Autodesk Fusion 360 part; units mm, degrees
(part 9 of 14)
  line L5619 (-23.7596, 111.125) -> (-29.2589, 101.6)
  line L5620 (-29.2589, 101.6) -> (-23.7596, 92.075)
  line L5621 (-23.7596, 92.075) -> (-12.7611, 92.075)
  line L5622 (-7.2618, 101.6) -> (-12.7611, 111.125)
  line L5623 (-12.7611, 92.075) -> (-7.2618, 101.6)
  line L5624 (6.4863, 122.2375) -> (-4.5122, 122.2375)
  line L5625 (-4.5122, 122.2375) -> (-10.0114, 112.7125)
  line L5626 (-10.0114, 112.7125) -> (-4.5122, 103.1875)
  line L5627 (-4.5122, 103.1875) -> (6.4863, 103.1875)
  line L5628 (11.9856, 112.7125) -> (6.4863, 122.2375)
  line L5629 (6.4863, 103.1875) -> (11.9856, 112.7125)
  line L5630 (25.7337, 133.35) -> (14.7352, 133.35)
  line L5631 (14.7352, 133.35) -> (9.236, 123.825)
  line L5632 (9.236, 123.825) -> (14.7352, 114.3)
  line L5633 (14.7352, 114.3) -> (25.7337, 114.3)
  line L5634 (31.233, 123.825) -> (25.7337, 133.35)
  line L5635 (25.7337, 114.3) -> (31.233, 123.825)
  line L5636 (44.9812, 144.4625) -> (33.9826, 144.4625)
  line L5637 (33.9826, 144.4625) -> (28.4834, 134.9375)
  line L5638 (28.4834, 134.9375) -> (33.9826, 125.4125)
  line L5639 (33.9826, 125.4125) -> (44.9812, 125.4125)
  line L5640 (50.4804, 134.9375) -> (44.9812, 144.4625)
  line L5641 (44.9812, 125.4125) -> (50.4804, 134.9375)
  line L5642 (64.2286, 155.575) -> (53.2301, 155.575)
  line L5643 (53.2301, 155.575) -> (47.7308, 146.05)
  line L5644 (47.7308, 146.05) -> (53.2301, 136.525)
  line L5645 (53.2301, 136.525) -> (64.2286, 136.525)
  line L5646 (69.7278, 146.05) -> (64.2286, 155.575)
  line L5647 (64.2286, 136.525) -> (69.7278, 146.05)
  line L5648 (83.476, 166.6875) -> (72.4775, 166.6875)
  line L5649 (72.4775, 166.6875) -> (66.9782, 157.1625)
  line L5650 (66.9782, 157.1625) -> (72.4775, 147.6375)
  line L5651 (72.4775, 147.6375) -> (83.476, 147.6375)
  line L5652 (88.9753, 157.1625) -> (83.476, 166.6875)
  line L5653 (83.476, 147.6375) -> (88.9753, 157.1625)
  line L5654 (102.7234, 177.8) -> (91.7249, 177.8)
  line L5655 (91.7249, 177.8) -> (86.2256, 168.275)
  line L5656 (86.2256, 168.275) -> (91.7249, 158.75)
  line L5657 (91.7249, 158.75) -> (102.7234, 158.75)
  line L5658 (108.2227, 168.275) -> (102.7234, 177.8)
  line L5659 (102.7234, 158.75) -> (108.2227, 168.275)
  line L5660 (121.9708, 188.9125) -> (110.9723, 188.9125)
  line L5661 (110.9723, 188.9125) -> (105.473, 179.3875)
  line L5662 (105.473, 179.3875) -> (110.9723, 169.8625)
  line L5663 (110.9723, 169.8625) -> (121.9708, 169.8625)
  line L5664 (127.4701, 179.3875) -> (121.9708, 188.9125)
  line L5665 (121.9708, 169.8625) -> (127.4701, 179.3875)
  line L5666 (141.2182, 200.025) -> (130.2197, 200.025)
  line L5667 (130.2197, 200.025) -> (124.7205, 190.5)
  line L5668 (124.7205, 190.5) -> (130.2197, 180.975)
  line L5669 (130.2197, 180.975) -> (141.2182, 180.975)
  line L5670 (146.7175, 190.5) -> (141.2182, 200.025)
  line L5671 (141.2182, 180.975) -> (146.7175, 190.5)
  line L5672 (160.4657, 211.1375) -> (149.4671, 211.1375)
  line L5673 (149.4671, 211.1375) -> (143.9679, 201.6125)
  line L5674 (143.9679, 201.6125) -> (149.4671, 192.0875)
  line L5675 (149.4671, 192.0875) -> (160.4657, 192.0875)
  line L5676 (165.9649, 201.6125) -> (160.4657, 211.1375)
  line L5677 (160.4657, 192.0875) -> (165.9649, 201.6125)
  line L5678 (179.7131, 222.25) -> (168.7145, 222.25)
  line L5679 (168.7145, 222.25) -> (163.2153, 212.725)
  line L5680 (163.2153, 212.725) -> (168.7145, 203.2)
  line L5681 (168.7145, 203.2) -> (179.7131, 203.2)
  line L5682 (185.2123, 212.725) -> (179.7131, 222.25)
  line L5683 (179.7131, 203.2) -> (185.2123, 212.725)
  line L5684 (198.9605, 233.3625) -> (187.962, 233.3625)
  line L5685 (187.962, 233.3625) -> (182.4627, 223.8375)
  line L5686 (182.4627, 223.8375) -> (187.962, 214.3125)
  line L5687 (187.962, 214.3125) -> (198.9605, 214.3125)
  line L5688 (204.4597, 223.8375) -> (198.9605, 233.3625)
  line L5689 (198.9605, 214.3125) -> (204.4597, 223.8375)
  line L5690 (218.2079, 244.475) -> (207.2094, 244.475)
  line L5691 (207.2094, 244.475) -> (201.7101, 234.95)
  line L5692 (201.7101, 234.95) -> (207.2094, 225.425)
  line L5693 (207.2094, 225.425) -> (218.2079, 225.425)
  line L5694 (223.7072, 234.95) -> (218.2079, 244.475)
  line L5695 (218.2079, 225.425) -> (223.7072, 234.95)
  line L5696 (237.4553, 255.5875) -> (226.4568, 255.5875)
  line L5697 (226.4568, 255.5875) -> (220.9575, 246.0625)
  line L5698 (220.9575, 246.0625) -> (226.4568, 236.5375)
  line L5699 (226.4568, 236.5375) -> (237.4553, 236.5375)
  line L5700 (242.9546, 246.0625) -> (237.4553, 255.5875)
  line L5701 (237.4553, 236.5375) -> (242.9546, 246.0625)
  line L5702 (256.7027, 266.7) -> (245.7042, 266.7)
  line L5703 (245.7042, 266.7) -> (240.2049, 257.175)
  line L5704 (240.2049, 257.175) -> (245.7042, 247.65)
  line L5705 (245.7042, 247.65) -> (256.7027, 247.65)
  line L5706 (262.202, 257.175) -> (256.7027, 266.7)
  line L5707 (256.7027, 247.65) -> (262.202, 257.175)
  line L5708 (275.9501, 277.8125) -> (264.9516, 277.8125)
  line L5709 (264.9516, 277.8125) -> (259.4524, 268.2875)
  line L5710 (259.4524, 268.2875) -> (264.9516, 258.7625)
  line L5711 (264.9516, 258.7625) -> (275.9501, 258.7625)
  line L5712 (281.4494, 268.2875) -> (275.9501, 277.8125)
  line L5713 (275.9501, 258.7625) -> (281.4494, 268.2875)
  line L5714 (295.1976, 288.925) -> (284.199, 288.925)
  line L5715 (284.199, 288.925) -> (278.6998, 279.4)
  line L5716 (278.6998, 279.4) -> (284.199, 269.875)
  line L5717 (284.199, 269.875) -> (295.1976, 269.875)
  line L5718 (300.6968, 279.4) -> (295.1976, 288.925)
  line L5719 (295.1976, 269.875) -> (300.6968, 279.4)
  line L5720 (314.445, 300.0375) -> (303.4464, 300.0375)
  line L5721 (303.4464, 300.0375) -> (297.9472, 290.5125)
  line L5722 (297.9472, 290.5125) -> (303.4464, 280.9875)
  line L5723 (303.4464, 280.9875) -> (314.445, 280.9875)
  line L5724 (319.9442, 290.5125) -> (314.445, 300.0375)
  line L5725 (314.445, 280.9875) -> (319.9442, 290.5125)
  line L5726 (333.6924, 311.15) -> (322.6939, 311.15)
  line L5727 (322.6939, 311.15) -> (317.1946, 301.625)
  line L5728 (317.1946, 301.625) -> (322.6939, 292.1)
  line L5729 (322.6939, 292.1) -> (333.6924, 292.1)
  line L5730 (339.1916, 301.625) -> (333.6924, 311.15)
  line L5731 (333.6924, 292.1) -> (339.1916, 301.625)
  line L5732 (352.9398, 322.2625) -> (341.9413, 322.2625)
  line L5733 (341.9413, 322.2625) -> (336.442, 312.7375)
  line L5734 (336.442, 312.7375) -> (341.9413, 303.2125)
  line L5735 (341.9413, 303.2125) -> (352.9398, 303.2125)
  line L5736 (358.4391, 312.7375) -> (352.9398, 322.2625)
  line L5737 (352.9398, 303.2125) -> (358.4391, 312.7375)
  line L5738 (372.1872, 333.375) -> (361.1887, 333.375)
  line L5739 (361.1887, 333.375) -> (355.6894, 323.85)
  line L5740 (355.6894, 323.85) -> (361.1887, 314.325)
  line L5741 (361.1887, 314.325) -> (372.1872, 314.325)
  line L5742 (377.6865, 323.85) -> (372.1872, 333.375)
  line L5743 (372.1872, 314.325) -> (377.6865, 323.85)
  line L5744 (391.4346, 344.4875) -> (380.4361, 344.4875)
  line L5745 (380.4361, 344.4875) -> (374.9368, 334.9625)
  line L5746 (374.9368, 334.9625) -> (380.4361, 325.4375)
  line L5747 (380.4361, 325.4375) -> (391.4346, 325.4375)
  line L5748 (396.9339, 334.9625) -> (391.4346, 344.4875)
  line L5749 (391.4346, 325.4375) -> (396.9339, 334.9625)
  line L5750 (410.682, 355.6) -> (399.6835, 355.6)
  line L5751 (399.6835, 355.6) -> (394.1843, 346.075)
  line L5752 (394.1843, 346.075) -> (399.6835, 336.55)
  line L5753 (399.6835, 336.55) -> (410.682, 336.55)
  line L5754 (416.1813, 346.075) -> (410.682, 355.6)
  line L5755 (410.682, 336.55) -> (416.1813, 346.075)
  line L5756 (429.9295, 366.7125) -> (418.9309, 366.7125)
  line L5757 (418.9309, 366.7125) -> (413.4317, 357.1875)
  line L5758 (413.4317, 357.1875) -> (418.9309, 347.6625)
  line L5759 (418.9309, 347.6625) -> (429.9295, 347.6625)
  line L5760 (435.4287, 357.1875) -> (429.9295, 366.7125)
  line L5761 (429.9295, 347.6625) -> (435.4287, 357.1875)
  line L5762 (449.1769, 377.825) -> (438.1783, 377.825)
  line L5763 (438.1783, 377.825) -> (432.6791, 368.3)
  line L5764 (432.6791, 368.3) -> (438.1783, 358.775)
  line L5765 (438.1783, 358.775) -> (449.1769, 358.775)
  line L5766 (454.6761, 368.3) -> (449.1769, 377.825)
  line L5767 (449.1769, 358.775) -> (454.6761, 368.3)
  line L5768 (468.4243, 388.9375) -> (457.4258, 388.9375)
  line L5769 (457.4258, 388.9375) -> (451.9265, 379.4125)
  line L5770 (451.9265, 379.4125) -> (457.4258, 369.8875)
  line L5771 (457.4258, 369.8875) -> (468.4243, 369.8875)
  line L5772 (473.9235, 379.4125) -> (468.4243, 388.9375)
  line L5773 (468.4243, 369.8875) -> (473.9235, 379.4125)
  line L5774 (-686.4206, -255.5875) -> (-697.4191, -255.5875)
  line L5775 (-697.4191, -255.5875) -> (-702.9184, -265.1125)
  line L5776 (-702.9184, -265.1125) -> (-697.4191, -274.6375)
  line L5777 (-697.4191, -274.6375) -> (-686.4206, -274.6375)
  line L5778 (-680.9213, -265.1125) -> (-686.4206, -255.5875)
  line L5779 (-686.4206, -274.6375) -> (-680.9213, -265.1125)
  line L5780 (-667.1732, -244.475) -> (-678.1717, -244.475)
  line L5781 (-678.1717, -244.475) -> (-683.671, -254)
  line L5782 (-683.671, -254) -> (-678.1717, -263.525)
  line L5783 (-678.1717, -263.525) -> (-667.1732, -263.525)
  line L5784 (-661.6739, -254) -> (-667.1732, -244.475)
  line L5785 (-667.1732, -263.525) -> (-661.6739, -254)
  line L5786 (-647.9258, -233.3625) -> (-658.9243, -233.3625)
  line L5787 (-658.9243, -233.3625) -> (-664.4235, -242.8875)
  line L5788 (-664.4235, -242.8875) -> (-658.9243, -252.4125)
  line L5789 (-658.9243, -252.4125) -> (-647.9258, -252.4125)
  line L5790 (-642.4265, -242.8875) -> (-647.9258, -233.3625)
  line L5791 (-647.9258, -252.4125) -> (-642.4265, -242.8875)
  line L5792 (-628.6783, -222.25) -> (-639.6769, -222.25)
  line L5793 (-639.6769, -222.25) -> (-645.1761, -231.775)
  line L5794 (-645.1761, -231.775) -> (-639.6769, -241.3)
  line L5795 (-639.6769, -241.3) -> (-628.6783, -241.3)
  line L5796 (-623.1791, -231.775) -> (-628.6783, -222.25)
  line L5797 (-628.6783, -241.3) -> (-623.1791, -231.775)
  line L5798 (-609.4309, -211.1375) -> (-620.4295, -211.1375)
  line L5799 (-620.4295, -211.1375) -> (-625.9287, -220.6625)
  line L5800 (-625.9287, -220.6625) -> (-620.4295, -230.1875)
  line L5801 (-620.4295, -230.1875) -> (-609.4309, -230.1875)
  line L5802 (-603.9317, -220.6625) -> (-609.4309, -211.1375)
  line L5803 (-609.4309, -230.1875) -> (-603.9317, -220.6625)
  line L5804 (-590.1835, -200.025) -> (-601.182, -200.025)
  line L5805 (-601.182, -200.025) -> (-606.6813, -209.55)
  line L5806 (-606.6813, -209.55) -> (-601.182, -219.075)
  line L5807 (-601.182, -219.075) -> (-590.1835, -219.075)
  line L5808 (-584.6843, -209.55) -> (-590.1835, -200.025)
  line L5809 (-590.1835, -219.075) -> (-584.6843, -209.55)
  line L5810 (-570.9361, -188.9125) -> (-581.9346, -188.9125)
  line L5811 (-581.9346, -188.9125) -> (-587.4339, -198.4375)
  line L5812 (-587.4339, -198.4375) -> (-581.9346, -207.9625)
  line L5813 (-581.9346, -207.9625) -> (-570.9361, -207.9625)
  line L5814 (-565.4368, -198.4375) -> (-570.9361, -188.9125)
  line L5815 (-570.9361, -207.9625) -> (-565.4368, -198.4375)
  line L5816 (-551.6887, -177.8) -> (-562.6872, -177.8)
  line L5817 (-562.6872, -177.8) -> (-568.1865, -187.325)
  line L5818 (-568.1865, -187.325) -> (-562.6872, -196.85)
  line L5819 (-562.6872, -196.85) -> (-551.6887, -196.85)
  line L5820 (-546.1894, -187.325) -> (-551.6887, -177.8)
  line L5821 (-551.6887, -196.85) -> (-546.1894, -187.325)
  line L5822 (-532.4413, -166.6875) -> (-543.4398, -166.6875)
  line L5823 (-543.4398, -166.6875) -> (-548.9391, -176.2125)
  line L5824 (-548.9391, -176.2125) -> (-543.4398, -185.7375)
  line L5825 (-543.4398, -185.7375) -> (-532.4413, -185.7375)
  line L5826 (-526.942, -176.2125) -> (-532.4413, -166.6875)
  line L5827 (-532.4413, -185.7375) -> (-526.942, -176.2125)
  line L5828 (-513.1939, -155.575) -> (-524.1924, -155.575)
  line L5829 (-524.1924, -155.575) -> (-529.6916, -165.1)
  line L5830 (-529.6916, -165.1) -> (-524.1924, -174.625)
  line L5831 (-524.1924, -174.625) -> (-513.1939, -174.625)
  line L5832 (-507.6946, -165.1) -> (-513.1939, -155.575)
  line L5833 (-513.1939, -174.625) -> (-507.6946, -165.1)
  line L5834 (-493.9464, -144.4625) -> (-504.945, -144.4625)
  line L5835 (-504.945, -144.4625) -> (-510.4442, -153.9875)
  line L5836 (-510.4442, -153.9875) -> (-504.945, -163.5125)
  line L5837 (-504.945, -163.5125) -> (-493.9464, -163.5125)
  line L5838 (-488.4472, -153.9875) -> (-493.9464, -144.4625)
  line L5839 (-493.9464, -163.5125) -> (-488.4472, -153.9875)
  line L5840 (-474.699, -133.35) -> (-485.6976, -133.35)
  line L5841 (-485.6976, -133.35) -> (-491.1968, -142.875)
  line L5842 (-491.1968, -142.875) -> (-485.6976, -152.4)
  line L5843 (-485.6976, -152.4) -> (-474.699, -152.4)
  line L5844 (-469.1998, -142.875) -> (-474.699, -133.35)
  line L5845 (-474.699, -152.4) -> (-469.1998, -142.875)
  line L5846 (-455.4516, -122.2375) -> (-466.4501, -122.2375)
  line L5847 (-466.4501, -122.2375) -> (-471.9494, -131.7625)
  line L5848 (-471.9494, -131.7625) -> (-466.4501, -141.2875)
  line L5849 (-466.4501, -141.2875) -> (-455.4516, -141.2875)
  line L5850 (-449.9524, -131.7625) -> (-455.4516, -122.2375)
  line L5851 (-455.4516, -141.2875) -> (-449.9524, -131.7625)
  line L5852 (-436.2042, -111.125) -> (-447.2027, -111.125)
  line L5853 (-447.2027, -111.125) -> (-452.702, -120.65)
  line L5854 (-452.702, -120.65) -> (-447.2027, -130.175)
  line L5855 (-447.2027, -130.175) -> (-436.2042, -130.175)
  line L5856 (-430.7049, -120.65) -> (-436.2042, -111.125)
  line L5857 (-436.2042, -130.175) -> (-430.7049, -120.65)
  line L5858 (-416.9568, -100.0125) -> (-427.9553, -100.0125)
  line L5859 (-427.9553, -100.0125) -> (-433.4546, -109.5375)
  line L5860 (-433.4546, -109.5375) -> (-427.9553, -119.0625)
  line L5861 (-427.9553, -119.0625) -> (-416.9568, -119.0625)
  line L5862 (-411.4575, -109.5375) -> (-416.9568, -100.0125)
  line L5863 (-416.9568, -119.0625) -> (-411.4575, -109.5375)
  line L5864 (-397.7094, -88.9) -> (-408.7079, -88.9)
  line L5865 (-408.7079, -88.9) -> (-414.2072, -98.425)
  line L5866 (-414.2072, -98.425) -> (-408.7079, -107.95)
  line L5867 (-408.7079, -107.95) -> (-397.7094, -107.95)
  line L5868 (-392.2101, -98.425) -> (-397.7094, -88.9)
  line L5869 (-397.7094, -107.95) -> (-392.2101, -98.425)
  line L5870 (-378.462, -77.7875) -> (-389.4605, -77.7875)
  line L5871 (-389.4605, -77.7875) -> (-394.9597, -87.3125)
  line L5872 (-394.9597, -87.3125) -> (-389.4605, -96.8375)
  line L5873 (-389.4605, -96.8375) -> (-378.462, -96.8375)
  line L5874 (-372.9627, -87.3125) -> (-378.462, -77.7875)
  line L5875 (-378.462, -96.8375) -> (-372.9627, -87.3125)
  line L5876 (-359.2145, -66.675) -> (-370.2131, -66.675)
  line L5877 (-370.2131, -66.675) -> (-375.7123, -76.2)
  line L5878 (-375.7123, -76.2) -> (-370.2131, -85.725)
  line L5879 (-370.2131, -85.725) -> (-359.2145, -85.725)
  line L5880 (-353.7153, -76.2) -> (-359.2145, -66.675)
  line L5881 (-359.2145, -85.725) -> (-353.7153, -76.2)
  line L5882 (-339.9671, -55.5625) -> (-350.9657, -55.5625)
  line L5883 (-350.9657, -55.5625) -> (-356.4649, -65.0875)
  line L5884 (-356.4649, -65.0875) -> (-350.9657, -74.6125)
  line L5885 (-350.9657, -74.6125) -> (-339.9671, -74.6125)
  line L5886 (-334.4679, -65.0875) -> (-339.9671, -55.5625)
  line L5887 (-339.9671, -74.6125) -> (-334.4679, -65.0875)
  line L5888 (-320.7197, -44.45) -> (-331.7182, -44.45)
  line L5889 (-331.7182, -44.45) -> (-337.2175, -53.975)
  line L5890 (-337.2175, -53.975) -> (-331.7182, -63.5)
  line L5891 (-331.7182, -63.5) -> (-320.7197, -63.5)
  line L5892 (-315.2205, -53.975) -> (-320.7197, -44.45)
  line L5893 (-320.7197, -63.5) -> (-315.2205, -53.975)
  line L5894 (-301.4723, -33.3375) -> (-312.4708, -33.3375)
  line L5895 (-312.4708, -33.3375) -> (-317.9701, -42.8625)
  line L5896 (-317.9701, -42.8625) -> (-312.4708, -52.3875)
  line L5897 (-312.4708, -52.3875) -> (-301.4723, -52.3875)
  line L5898 (-295.973, -42.8625) -> (-301.4723, -33.3375)
  line L5899 (-301.4723, -52.3875) -> (-295.973, -42.8625)
  line L5900 (-282.2249, -22.225) -> (-293.2234, -22.225)
  line L5901 (-293.2234, -22.225) -> (-298.7227, -31.75)
  line L5902 (-298.7227, -31.75) -> (-293.2234, -41.275)
  line L5903 (-293.2234, -41.275) -> (-282.2249, -41.275)
  line L5904 (-276.7256, -31.75) -> (-282.2249, -22.225)
  line L5905 (-282.2249, -41.275) -> (-276.7256, -31.75)
  line L5906 (-262.9775, -11.1125) -> (-273.976, -11.1125)
  line L5907 (-273.976, -11.1125) -> (-279.4753, -20.6375)
  line L5908 (-279.4753, -20.6375) -> (-273.976, -30.1625)
  line L5909 (-273.976, -30.1625) -> (-262.9775, -30.1625)
  line L5910 (-257.4782, -20.6375) -> (-262.9775, -11.1125)
  line L5911 (-262.9775, -30.1625) -> (-257.4782, -20.6375)
  line L5912 (-243.7301, 0) -> (-254.7286, 0)
  line L5913 (-254.7286, 0) -> (-260.2278, -9.525)
  line L5914 (-260.2278, -9.525) -> (-254.7286, -19.05)
  line L5915 (-254.7286, -19.05) -> (-243.7301, -19.05)
  line L5916 (-238.2308, -9.525) -> (-243.7301, 0)
  line L5917 (-243.7301, -19.05) -> (-238.2308, -9.525)
  line L5918 (-224.4826, 11.1125) -> (-235.4812, 11.1125)
  line L5919 (-235.4812, 11.1125) -> (-240.9804, 1.5875)
  line L5920 (-240.9804, 1.5875) -> (-235.4812, -7.9375)
  line L5921 (-235.4812, -7.9375) -> (-224.4826, -7.9375)
  line L5922 (-218.9834, 1.5875) -> (-224.4826, 11.1125)
  line L5923 (-224.4826, -7.9375) -> (-218.9834, 1.5875)
  line L5924 (-205.2352, 22.225) -> (-216.2337, 22.225)
  line L5925 (-216.2337, 22.225) -> (-221.733, 12.7)
  line L5926 (-221.733, 12.7) -> (-216.2337, 3.175)
  line L5927 (-216.2337, 3.175) -> (-205.2352, 3.175)
  line L5928 (-199.736, 12.7) -> (-205.2352, 22.225)
  line L5929 (-205.2352, 3.175) -> (-199.736, 12.7)
  line L5930 (-185.9878, 33.3375) -> (-196.9863, 33.3375)
  line L5931 (-196.9863, 33.3375) -> (-202.4856, 23.8125)
  line L5932 (-202.4856, 23.8125) -> (-196.9863, 14.2875)
  line L5933 (-196.9863, 14.2875) -> (-185.9878, 14.2875)
  line L5934 (-180.4886, 23.8125) -> (-185.9878, 33.3375)
  line L5935 (-185.9878, 14.2875) -> (-180.4886, 23.8125)
  line L5936 (-166.7404, 44.45) -> (-177.7389, 44.45)
  line L5937 (-177.7389, 44.45) -> (-183.2382, 34.925)
  line L5938 (-183.2382, 34.925) -> (-177.7389, 25.4)
  line L5939 (-177.7389, 25.4) -> (-166.7404, 25.4)
  line L5940 (-161.2411, 34.925) -> (-166.7404, 44.45)
  line L5941 (-166.7404, 25.4) -> (-161.2411, 34.925)
  line L5942 (-147.493, 55.5625) -> (-158.4915, 55.5625)
  line L5943 (-158.4915, 55.5625) -> (-163.9908, 46.0375)
  line L5944 (-163.9908, 46.0375) -> (-158.4915, 36.5125)
  line L5945 (-158.4915, 36.5125) -> (-147.493, 36.5125)
  line L5946 (-141.9937, 46.0375) -> (-147.493, 55.5625)
  line L5947 (-147.493, 36.5125) -> (-141.9937, 46.0375)
  line L5948 (-128.2456, 66.675) -> (-139.2441, 66.675)
  line L5949 (-139.2441, 66.675) -> (-144.7434, 57.15)
  line L5950 (-144.7434, 57.15) -> (-139.2441, 47.625)
  line L5951 (-139.2441, 47.625) -> (-128.2456, 47.625)
  line L5952 (-122.7463, 57.15) -> (-128.2456, 66.675)
  line L5953 (-128.2456, 47.625) -> (-122.7463, 57.15)
  line L5954 (-108.9982, 77.7875) -> (-119.9967, 77.7875)
  line L5955 (-119.9967, 77.7875) -> (-125.4959, 68.2625)
  line L5956 (-125.4959, 68.2625) -> (-119.9967, 58.7375)
  line L5957 (-119.9967, 58.7375) -> (-108.9982, 58.7375)
  line L5958 (-103.4989, 68.2625) -> (-108.9982, 77.7875)
  line L5959 (-108.9982, 58.7375) -> (-103.4989, 68.2625)
  line L5960 (-89.7507, 88.9) -> (-100.7493, 88.9)
  line L5961 (-100.7493, 88.9) -> (-106.2485, 79.375)
  line L5962 (-106.2485, 79.375) -> (-100.7493, 69.85)
  line L5963 (-100.7493, 69.85) -> (-89.7507, 69.85)
  line L5964 (-84.2515, 79.375) -> (-89.7507, 88.9)
  line L5965 (-89.7507, 69.85) -> (-84.2515, 79.375)
  line L5966 (-70.5033, 100.0125) -> (-81.5018, 100.0125)
  line L5967 (-81.5018, 100.0125) -> (-87.0011, 90.4875)
  line L5968 (-87.0011, 90.4875) -> (-81.5018, 80.9625)
  line L5969 (-81.5018, 80.9625) -> (-70.5033, 80.9625)
  line L5970 (-65.0041, 90.4875) -> (-70.5033, 100.0125)
  line L5971 (-70.5033, 80.9625) -> (-65.0041, 90.4875)
  line L5972 (-51.2559, 111.125) -> (-62.2544, 111.125)
  line L5973 (-62.2544, 111.125) -> (-67.7537, 101.6)
  line L5974 (-67.7537, 101.6) -> (-62.2544, 92.075)
  line L5975 (-62.2544, 92.075) -> (-51.2559, 92.075)
  line L5976 (-45.7566, 101.6) -> (-51.2559, 111.125)
  line L5977 (-51.2559, 92.075) -> (-45.7566, 101.6)
  line L5978 (-32.0085, 122.2375) -> (-43.007, 122.2375)
  line L5979 (-43.007, 122.2375) -> (-48.5063, 112.7125)
  line L5980 (-48.5063, 112.7125) -> (-43.007, 103.1875)
  line L5981 (-43.007, 103.1875) -> (-32.0085, 103.1875)
  line L5982 (-26.5092, 112.7125) -> (-32.0085, 122.2375)
  line L5983 (-32.0085, 103.1875) -> (-26.5092, 112.7125)
  line L5984 (-12.7611, 133.35) -> (-23.7596, 133.35)
  line L5985 (-23.7596, 133.35) -> (-29.2589, 123.825)
  line L5986 (-29.2589, 123.825) -> (-23.7596, 114.3)
  line L5987 (-23.7596, 114.3) -> (-12.7611, 114.3)
  line L5988 (-7.2618, 123.825) -> (-12.7611, 133.35)
  line L5989 (-12.7611, 114.3) -> (-7.2618, 123.825)
  line L5990 (6.4863, 144.4625) -> (-4.5122, 144.4625)
  line L5991 (-4.5122, 144.4625) -> (-10.0114, 134.9375)
  line L5992 (-10.0114, 134.9375) -> (-4.5122, 125.4125)
  line L5993 (-4.5122, 125.4125) -> (6.4863, 125.4125)
  line L5994 (11.9856, 134.9375) -> (6.4863, 144.4625)
  line L5995 (6.4863, 125.4125) -> (11.9856, 134.9375)
  line L5996 (25.7337, 155.575) -> (14.7352, 155.575)
  line L5997 (14.7352, 155.575) -> (9.236, 146.05)
  line L5998 (9.236, 146.05) -> (14.7352, 136.525)
  line L5999 (14.7352, 136.525) -> (25.7337, 136.525)
  line L6000 (31.233, 146.05) -> (25.7337, 155.575)
  line L6001 (25.7337, 136.525) -> (31.233, 146.05)
  line L6002 (44.9812, 166.6875) -> (33.9826, 166.6875)
  line L6003 (33.9826, 166.6875) -> (28.4834, 157.1625)
  line L6004 (28.4834, 157.1625) -> (33.9826, 147.6375)
  line L6005 (33.9826, 147.6375) -> (44.9812, 147.6375)
  line L6006 (50.4804, 157.1625) -> (44.9812, 166.6875)
  line L6007 (44.9812, 147.6375) -> (50.4804, 157.1625)
  line L6008 (64.2286, 177.8) -> (53.2301, 177.8)
  line L6009 (53.2301, 177.8) -> (47.7308, 168.275)
  line L6010 (47.7308, 168.275) -> (53.2301, 158.75)
  line L6011 (53.2301, 158.75) -> (64.2286, 158.75)
  line L6012 (69.7278, 168.275) -> (64.2286, 177.8)
  line L6013 (64.2286, 158.75) -> (69.7278, 168.275)
  line L6014 (83.476, 188.9125) -> (72.4775, 188.9125)
  line L6015 (72.4775, 188.9125) -> (66.9782, 179.3875)
  line L6016 (66.9782, 179.3875) -> (72.4775, 169.8625)
  line L6017 (72.4775, 169.8625) -> (83.476, 169.8625)
  line L6018 (88.9753, 179.3875) -> (83.476, 188.9125)
  line L6019 (83.476, 169.8625) -> (88.9753, 179.3875)
  line L6020 (102.7234, 200.025) -> (91.7249, 200.025)
  line L6021 (91.7249, 200.025) -> (86.2256, 190.5)
  line L6022 (86.2256, 190.5) -> (91.7249, 180.975)
  line L6023 (91.7249, 180.975) -> (102.7234, 180.975)
  line L6024 (108.2227, 190.5) -> (102.7234, 200.025)
  line L6025 (102.7234, 180.975) -> (108.2227, 190.5)
  line L6026 (121.9708, 211.1375) -> (110.9723, 211.1375)
  line L6027 (110.9723, 211.1375) -> (105.473, 201.6125)
  line L6028 (105.473, 201.6125) -> (110.9723, 192.0875)
  line L6029 (110.9723, 192.0875) -> (121.9708, 192.0875)
  line L6030 (127.4701, 201.6125) -> (121.9708, 211.1375)
  line L6031 (121.9708, 192.0875) -> (127.4701, 201.6125)
  line L6032 (141.2182, 222.25) -> (130.2197, 222.25)
  line L6033 (130.2197, 222.25) -> (124.7205, 212.725)
  line L6034 (124.7205, 212.725) -> (130.2197, 203.2)
  line L6035 (130.2197, 203.2) -> (141.2182, 203.2)
  line L6036 (146.7175, 212.725) -> (141.2182, 222.25)
  line L6037 (141.2182, 203.2) -> (146.7175, 212.725)
  line L6038 (160.4657, 233.3625) -> (149.4671, 233.3625)
  line L6039 (149.4671, 233.3625) -> (143.9679, 223.8375)
  line L6040 (143.9679, 223.8375) -> (149.4671, 214.3125)
  line L6041 (149.4671, 214.3125) -> (160.4657, 214.3125)
  line L6042 (165.9649, 223.8375) -> (160.4657, 233.3625)
  line L6043 (160.4657, 214.3125) -> (165.9649, 223.8375)
  line L6044 (179.7131, 244.475) -> (168.7145, 244.475)
  line L6045 (168.7145, 244.475) -> (163.2153, 234.95)
  line L6046 (163.2153, 234.95) -> (168.7145, 225.425)
  line L6047 (168.7145, 225.425) -> (179.7131, 225.425)
  line L6048 (185.2123, 234.95) -> (179.7131, 244.475)
  line L6049 (179.7131, 225.425) -> (185.2123, 234.95)
  line L6050 (198.9605, 255.5875) -> (187.962, 255.5875)
  line L6051 (187.962, 255.5875) -> (182.4627, 246.0625)
  line L6052 (182.4627, 246.0625) -> (187.962, 236.5375)
  line L6053 (187.962, 236.5375) -> (198.9605, 236.5375)
  line L6054 (204.4597, 246.0625) -> (198.9605, 255.5875)
  line L6055 (198.9605, 236.5375) -> (204.4597, 246.0625)
  line L6056 (218.2079, 266.7) -> (207.2094, 266.7)
  line L6057 (207.2094, 266.7) -> (201.7101, 257.175)
  line L6058 (201.7101, 257.175) -> (207.2094, 247.65)
  line L6059 (207.2094, 247.65) -> (218.2079, 247.65)
  line L6060 (223.7072, 257.175) -> (218.2079, 266.7)
  line L6061 (218.2079, 247.65) -> (223.7072, 257.175)
  line L6062 (237.4553, 277.8125) -> (226.4568, 277.8125)
  line L6063 (226.4568, 277.8125) -> (220.9575, 268.2875)
  line L6064 (220.9575, 268.2875) -> (226.4568, 258.7625)
  line L6065 (226.4568, 258.7625) -> (237.4553, 258.7625)
  line L6066 (242.9546, 268.2875) -> (237.4553, 277.8125)
  line L6067 (237.4553, 258.7625) -> (242.9546, 268.2875)
  line L6068 (256.7027, 288.925) -> (245.7042, 288.925)
  line L6069 (245.7042, 288.925) -> (240.2049, 279.4)
  line L6070 (240.2049, 279.4) -> (245.7042, 269.875)
  line L6071 (245.7042, 269.875) -> (256.7027, 269.875)
  line L6072 (262.202, 279.4) -> (256.7027, 288.925)
  line L6073 (256.7027, 269.875) -> (262.202, 279.4)
  line L6074 (275.9501, 300.0375) -> (264.9516, 300.0375)
  line L6075 (264.9516, 300.0375) -> (259.4524, 290.5125)
  line L6076 (259.4524, 290.5125) -> (264.9516, 280.9875)
  line L6077 (264.9516, 280.9875) -> (275.9501, 280.9875)
  line L6078 (281.4494, 290.5125) -> (275.9501, 300.0375)
  line L6079 (275.9501, 280.9875) -> (281.4494, 290.5125)
  line L6080 (295.1976, 311.15) -> (284.199, 311.15)
  line L6081 (284.199, 311.15) -> (278.6998, 301.625)
  line L6082 (278.6998, 301.625) -> (284.199, 292.1)
  line L6083 (284.199, 292.1) -> (295.1976, 292.1)
  line L6084 (300.6968, 301.625) -> (295.1976, 311.15)
  line L6085 (295.1976, 292.1) -> (300.6968, 301.625)
  line L6086 (314.445, 322.2625) -> (303.4464, 322.2625)
  line L6087 (303.4464, 322.2625) -> (297.9472, 312.7375)
  line L6088 (297.9472, 312.7375) -> (303.4464, 303.2125)
  line L6089 (303.4464, 303.2125) -> (314.445, 303.2125)
  line L6090 (319.9442, 312.7375) -> (314.445, 322.2625)
  line L6091 (314.445, 303.2125) -> (319.9442, 312.7375)
  line L6092 (333.6924, 333.375) -> (322.6939, 333.375)
  line L6093 (322.6939, 333.375) -> (317.1946, 323.85)
  line L6094 (317.1946, 323.85) -> (322.6939, 314.325)
  line L6095 (322.6939, 314.325) -> (333.6924, 314.325)
  line L6096 (339.1916, 323.85) -> (333.6924, 333.375)
  line L6097 (333.6924, 314.325) -> (339.1916, 323.85)
  line L6098 (352.9398, 344.4875) -> (341.9413, 344.4875)
  line L6099 (341.9413, 344.4875) -> (336.442, 334.9625)
  line L6100 (336.442, 334.9625) -> (341.9413, 325.4375)
  line L6101 (341.9413, 325.4375) -> (352.9398, 325.4375)
  line L6102 (358.4391, 334.9625) -> (352.9398, 344.4875)
  line L6103 (352.9398, 325.4375) -> (358.4391, 334.9625)
  line L6104 (372.1872, 355.6) -> (361.1887, 355.6)
  line L6105 (361.1887, 355.6) -> (355.6894, 346.075)
  line L6106 (355.6894, 346.075) -> (361.1887, 336.55)
  line L6107 (361.1887, 336.55) -> (372.1872, 336.55)
  line L6108 (377.6865, 346.075) -> (372.1872, 355.6)
  line L6109 (372.1872, 336.55) -> (377.6865, 346.075)
  line L6110 (391.4346, 366.7125) -> (380.4361, 366.7125)
  line L6111 (380.4361, 366.7125) -> (374.9368, 357.1875)
  line L6112 (374.9368, 357.1875) -> (380.4361, 347.6625)
  line L6113 (380.4361, 347.6625) -> (391.4346, 347.6625)
  line L6114 (396.9339, 357.1875) -> (391.4346, 366.7125)
  line L6115 (391.4346, 347.6625) -> (396.9339, 357.1875)
  line L6116 (410.682, 377.825) -> (399.6835, 377.825)
  line L6117 (399.6835, 377.825) -> (394.1843, 368.3)
  line L6118 (394.1843, 368.3) -> (399.6835, 358.775)
  line L6119 (399.6835, 358.775) -> (410.682, 358.775)
  line L6120 (416.1813, 368.3) -> (410.682, 377.825)
  line L6121 (410.682, 358.775) -> (416.1813, 368.3)
  line L6122 (429.9295, 388.9375) -> (418.9309, 388.9375)
  line L6123 (418.9309, 388.9375) -> (413.4317, 379.4125)
  line L6124 (413.4317, 379.4125) -> (418.9309, 369.8875)
  line L6125 (418.9309, 369.8875) -> (429.9295, 369.8875)
  line L6126 (435.4287, 379.4125) -> (429.9295, 388.9375)
  line L6127 (429.9295, 369.8875) -> (435.4287, 379.4125)
  line L6128 (449.1769, 400.05) -> (438.1783, 400.05)
  line L6129 (438.1783, 400.05) -> (432.6791, 390.525)
  line L6130 (432.6791, 390.525) -> (438.1783, 381)
  line L6131 (438.1783, 381) -> (449.1769, 381)
  line L6132 (454.6761, 390.525) -> (449.1769, 400.05)
  line L6133 (449.1769, 381) -> (454.6761, 390.525)
  line L6134 (-705.668, -244.475) -> (-716.6665, -244.475)
  line L6135 (-716.6665, -244.475) -> (-722.1658, -254)
  line L6136 (-722.1658, -254) -> (-716.6665, -263.525)
  line L6137 (-716.6665, -263.525) -> (-705.668, -263.525)
  line L6138 (-700.1687, -254) -> (-705.668, -244.475)
  line L6139 (-705.668, -263.525) -> (-700.1687, -254)
  line L6140 (-686.4206, -233.3625) -> (-697.4191, -233.3625)
  line L6141 (-697.4191, -233.3625) -> (-702.9184, -242.8875)
  line L6142 (-702.9184, -242.8875) -> (-697.4191, -252.4125)
  line L6143 (-697.4191, -252.4125) -> (-686.4206, -252.4125)
  line L6144 (-680.9213, -242.8875) -> (-686.4206, -233.3625)
  line L6145 (-686.4206, -252.4125) -> (-680.9213, -242.8875)
  line L6146 (-667.1732, -222.25) -> (-678.1717, -222.25)
  line L6147 (-678.1717, -222.25) -> (-683.671, -231.775)
  line L6148 (-683.671, -231.775) -> (-678.1717, -241.3)
  line L6149 (-678.1717, -241.3) -> (-667.1732, -241.3)
  line L6150 (-661.6739, -231.775) -> (-667.1732, -222.25)
  line L6151 (-667.1732, -241.3) -> (-661.6739, -231.775)
  line L6152 (-647.9258, -211.1375) -> (-658.9243, -211.1375)
  line L6153 (-658.9243, -211.1375) -> (-664.4235, -220.6625)
  line L6154 (-664.4235, -220.6625) -> (-658.9243, -230.1875)
  line L6155 (-658.9243, -230.1875) -> (-647.9258, -230.1875)
  line L6156 (-642.4265, -220.6625) -> (-647.9258, -211.1375)
  line L6157 (-647.9258, -230.1875) -> (-642.4265, -220.6625)
  line L6158 (-628.6783, -200.025) -> (-639.6769, -200.025)
  line L6159 (-639.6769, -200.025) -> (-645.1761, -209.55)
  line L6160 (-645.1761, -209.55) -> (-639.6769, -219.075)
  line L6161 (-639.6769, -219.075) -> (-628.6783, -219.075)
  line L6162 (-623.1791, -209.55) -> (-628.6783, -200.025)
  line L6163 (-628.6783, -219.075) -> (-623.1791, -209.55)
  line L6164 (-609.4309, -188.9125) -> (-620.4295, -188.9125)
  line L6165 (-620.4295, -188.9125) -> (-625.9287, -198.4375)
  line L6166 (-625.9287, -198.4375) -> (-620.4295, -207.9625)
  line L6167 (-620.4295, -207.9625) -> (-609.4309, -207.9625)
  line L6168 (-603.9317, -198.4375) -> (-609.4309, -188.9125)
  line L6169 (-609.4309, -207.9625) -> (-603.9317, -198.4375)
  line L6170 (-590.1835, -177.8) -> (-601.182, -177.8)
  line L6171 (-601.182, -177.8) -> (-606.6813, -187.325)
  line L6172 (-606.6813, -187.325) -> (-601.182, -196.85)
  line L6173 (-601.182, -196.85) -> (-590.1835, -196.85)
  line L6174 (-584.6843, -187.325) -> (-590.1835, -177.8)
  line L6175 (-590.1835, -196.85) -> (-584.6843, -187.325)
  line L6176 (-570.9361, -166.6875) -> (-581.9346, -166.6875)
  line L6177 (-581.9346, -166.6875) -> (-587.4339, -176.2125)
  line L6178 (-587.4339, -176.2125) -> (-581.9346, -185.7375)
  line L6179 (-581.9346, -185.7375) -> (-570.9361, -185.7375)
  line L6180 (-565.4368, -176.2125) -> (-570.9361, -166.6875)
  line L6181 (-570.9361, -185.7375) -> (-565.4368, -176.2125)
  line L6182 (-551.6887, -155.575) -> (-562.6872, -155.575)
  line L6183 (-562.6872, -155.575) -> (-568.1865, -165.1)
  line L6184 (-568.1865, -165.1) -> (-562.6872, -174.625)
  line L6185 (-562.6872, -174.625) -> (-551.6887, -174.625)
  line L6186 (-546.1894, -165.1) -> (-551.6887, -155.575)
  line L6187 (-551.6887, -174.625) -> (-546.1894, -165.1)
  line L6188 (-532.4413, -144.4625) -> (-543.4398, -144.4625)
  line L6189 (-543.4398, -144.4625) -> (-548.9391, -153.9875)
  line L6190 (-548.9391, -153.9875) -> (-543.4398, -163.5125)
  line L6191 (-543.4398, -163.5125) -> (-532.4413, -163.5125)
  line L6192 (-526.942, -153.9875) -> (-532.4413, -144.4625)
  line L6193 (-532.4413, -163.5125) -> (-526.942, -153.9875)
  line L6194 (-513.1939, -133.35) -> (-524.1924, -133.35)
  line L6195 (-524.1924, -133.35) -> (-529.6916, -142.875)
  line L6196 (-529.6916, -142.875) -> (-524.1924, -152.4)
  line L6197 (-524.1924, -152.4) -> (-513.1939, -152.4)
  line L6198 (-507.6946, -142.875) -> (-513.1939, -133.35)
  line L6199 (-513.1939, -152.4) -> (-507.6946, -142.875)
  line L6200 (-493.9464, -122.2375) -> (-504.945, -122.2375)
  line L6201 (-504.945, -122.2375) -> (-510.4442, -131.7625)
  line L6202 (-510.4442, -131.7625) -> (-504.945, -141.2875)
  line L6203 (-504.945, -141.2875) -> (-493.9464, -141.2875)
  line L6204 (-488.4472, -131.7625) -> (-493.9464, -122.2375)
  line L6205 (-493.9464, -141.2875) -> (-488.4472, -131.7625)
  line L6206 (-474.699, -111.125) -> (-485.6976, -111.125)
  line L6207 (-485.6976, -111.125) -> (-491.1968, -120.65)
  line L6208 (-491.1968, -120.65) -> (-485.6976, -130.175)
  line L6209 (-485.6976, -130.175) -> (-474.699, -130.175)
  line L6210 (-469.1998, -120.65) -> (-474.699, -111.125)
  line L6211 (-474.699, -130.175) -> (-469.1998, -120.65)
  line L6212 (-455.4516, -100.0125) -> (-466.4501, -100.0125)
  line L6213 (-466.4501, -100.0125) -> (-471.9494, -109.5375)
  line L6214 (-471.9494, -109.5375) -> (-466.4501, -119.0625)
  line L6215 (-466.4501, -119.0625) -> (-455.4516, -119.0625)
  line L6216 (-449.9524, -109.5375) -> (-455.4516, -100.0125)
  line L6217 (-455.4516, -119.0625) -> (-449.9524, -109.5375)
  line L6218 (-436.2042, -88.9) -> (-447.2027, -88.9)
  line L6219 (-447.2027, -88.9) -> (-452.702, -98.425)
  line L6220 (-452.702, -98.425) -> (-447.2027, -107.95)
  line L6221 (-447.2027, -107.95) -> (-436.2042, -107.95)
  line L6222 (-430.7049, -98.425) -> (-436.2042, -88.9)
  line L6223 (-436.2042, -107.95) -> (-430.7049, -98.425)
  line L6224 (-416.9568, -77.7875) -> (-427.9553, -77.7875)
  line L6225 (-427.9553, -77.7875) -> (-433.4546, -87.3125)
  line L6226 (-433.4546, -87.3125) -> (-427.9553, -96.8375)
  line L6227 (-427.9553, -96.8375) -> (-416.9568, -96.8375)
  line L6228 (-411.4575, -87.3125) -> (-416.9568, -77.7875)
  line L6229 (-416.9568, -96.8375) -> (-411.4575, -87.3125)
  line L6230 (-397.7094, -66.675) -> (-408.7079, -66.675)
  line L6231 (-408.7079, -66.675) -> (-414.2072, -76.2)
  line L6232 (-414.2072, -76.2) -> (-408.7079, -85.725)
  line L6233 (-408.7079, -85.725) -> (-397.7094, -85.725)
  line L6234 (-392.2101, -76.2) -> (-397.7094, -66.675)
  line L6235 (-397.7094, -85.725) -> (-392.2101, -76.2)
  line L6236 (-378.462, -55.5625) -> (-389.4605, -55.5625)
  line L6237 (-389.4605, -55.5625) -> (-394.9597, -65.0875)
  line L6238 (-394.9597, -65.0875) -> (-389.4605, -74.6125)
  line L6239 (-389.4605, -74.6125) -> (-378.462, -74.6125)
  line L6240 (-372.9627, -65.0875) -> (-378.462, -55.5625)
  line L6241 (-378.462, -74.6125) -> (-372.9627, -65.0875)
  line L6242 (-359.2145, -44.45) -> (-370.2131, -44.45)
  line L6243 (-370.2131, -44.45) -> (-375.7123, -53.975)
  line L6244 (-375.7123, -53.975) -> (-370.2131, -63.5)
  line L6245 (-370.2131, -63.5) -> (-359.2145, -63.5)
  line L6246 (-353.7153, -53.975) -> (-359.2145, -44.45)
  line L6247 (-359.2145, -63.5) -> (-353.7153, -53.975)
  line L6248 (-339.9671, -33.3375) -> (-350.9657, -33.3375)
  line L6249 (-350.9657, -33.3375) -> (-356.4649, -42.8625)
  line L6250 (-356.4649, -42.8625) -> (-350.9657, -52.3875)
  line L6251 (-350.9657, -52.3875) -> (-339.9671, -52.3875)
  line L6252 (-334.4679, -42.8625) -> (-339.9671, -33.3375)
  line L6253 (-339.9671, -52.3875) -> (-334.4679, -42.8625)
  line L6254 (-320.7197, -22.225) -> (-331.7182, -22.225)
  line L6255 (-331.7182, -22.225) -> (-337.2175, -31.75)
  line L6256 (-337.2175, -31.75) -> (-331.7182, -41.275)
  line L6257 (-331.7182, -41.275) -> (-320.7197, -41.275)
  line L6258 (-315.2205, -31.75) -> (-320.7197, -22.225)
  line L6259 (-320.7197, -41.275) -> (-315.2205, -31.75)
  line L6260 (-301.4723, -11.1125) -> (-312.4708, -11.1125)
  line L6261 (-312.4708, -11.1125) -> (-317.9701, -20.6375)
  line L6262 (-317.9701, -20.6375) -> (-312.4708, -30.1625)
  line L6263 (-312.4708, -30.1625) -> (-301.4723, -30.1625)
  line L6264 (-295.973, -20.6375) -> (-301.4723, -11.1125)
  line L6265 (-301.4723, -30.1625) -> (-295.973, -20.6375)
  line L6266 (-282.2249, 0) -> (-293.2234, 0)
  line L6267 (-293.2234, 0) -> (-298.7227, -9.525)
  line L6268 (-298.7227, -9.525) -> (-293.2234, -19.05)
  line L6269 (-293.2234, -19.05) -> (-282.2249, -19.05)
  line L6270 (-276.7256, -9.525) -> (-282.2249, 0)
  line L6271 (-282.2249, -19.05) -> (-276.7256, -9.525)
  line L6272 (-262.9775, 11.1125) -> (-273.976, 11.1125)
  line L6273 (-273.976, 11.1125) -> (-279.4753, 1.5875)
  line L6274 (-279.4753, 1.5875) -> (-273.976, -7.9375)
  line L6275 (-273.976, -7.9375) -> (-262.9775, -7.9375)
  line L6276 (-257.4782, 1.5875) -> (-262.9775, 11.1125)
  line L6277 (-262.9775, -7.9375) -> (-257.4782, 1.5875)
  line L6278 (-243.7301, 22.225) -> (-254.7286, 22.225)
  line L6279 (-254.7286, 22.225) -> (-260.2278, 12.7)
  line L6280 (-260.2278, 12.7) -> (-254.7286, 3.175)
  line L6281 (-254.7286, 3.175) -> (-243.7301, 3.175)
  line L6282 (-238.2308, 12.7) -> (-243.7301, 22.225)
  line L6283 (-243.7301, 3.175) -> (-238.2308, 12.7)
  line L6284 (-224.4826, 33.3375) -> (-235.4812, 33.3375)
  line L6285 (-235.4812, 33.3375) -> (-240.9804, 23.8125)
  line L6286 (-240.9804, 23.8125) -> (-235.4812, 14.2875)
  line L6287 (-235.4812, 14.2875) -> (-224.4826, 14.2875)
  line L6288 (-218.9834, 23.8125) -> (-224.4826, 33.3375)
  line L6289 (-224.4826, 14.2875) -> (-218.9834, 23.8125)
  line L6290 (-205.2352, 44.45) -> (-216.2337, 44.45)
  line L6291 (-216.2337, 44.45) -> (-221.733, 34.925)
  line L6292 (-221.733, 34.925) -> (-216.2337, 25.4)
  line L6293 (-216.2337, 25.4) -> (-205.2352, 25.4)
  line L6294 (-199.736, 34.925) -> (-205.2352, 44.45)
  line L6295 (-205.2352, 25.4) -> (-199.736, 34.925)
  line L6296 (-185.9878, 55.5625) -> (-196.9863, 55.5625)
  line L6297 (-196.9863, 55.5625) -> (-202.4856, 46.0375)
  line L6298 (-202.4856, 46.0375) -> (-196.9863, 36.5125)
  line L6299 (-196.9863, 36.5125) -> (-185.9878, 36.5125)
  line L6300 (-180.4886, 46.0375) -> (-185.9878, 55.5625)
  line L6301 (-185.9878, 36.5125) -> (-180.4886, 46.0375)
  line L6302 (-166.7404, 66.675) -> (-177.7389, 66.675)
  line L6303 (-177.7389, 66.675) -> (-183.2382, 57.15)
  line L6304 (-183.2382, 57.15) -> (-177.7389, 47.625)
  line L6305 (-177.7389, 47.625) -> (-166.7404, 47.625)
  line L6306 (-161.2411, 57.15) -> (-166.7404, 66.675)
  line L6307 (-166.7404, 47.625) -> (-161.2411, 57.15)
  line L6308 (-147.493, 77.7875) -> (-158.4915, 77.7875)
  line L6309 (-158.4915, 77.7875) -> (-163.9908, 68.2625)
  line L6310 (-163.9908, 68.2625) -> (-158.4915, 58.7375)
  line L6311 (-158.4915, 58.7375) -> (-147.493, 58.7375)
  line L6312 (-141.9937, 68.2625) -> (-147.493, 77.7875)
  line L6313 (-147.493, 58.7375) -> (-141.9937, 68.2625)
  line L6314 (-128.2456, 88.9) -> (-139.2441, 88.9)
  line L6315 (-139.2441, 88.9) -> (-144.7434, 79.375)
  line L6316 (-144.7434, 79.375) -> (-139.2441, 69.85)
  line L6317 (-139.2441, 69.85) -> (-128.2456, 69.85)
  line L6318 (-122.7463, 79.375) -> (-128.2456, 88.9)
  line L6319 (-128.2456, 69.85) -> (-122.7463, 79.375)
  line L6320 (-108.9982, 100.0125) -> (-119.9967, 100.0125)
  line L6321 (-119.9967, 100.0125) -> (-125.4959, 90.4875)
  line L6322 (-125.4959, 90.4875) -> (-119.9967, 80.9625)
  line L6323 (-119.9967, 80.9625) -> (-108.9982, 80.9625)
  line L6324 (-103.4989, 90.4875) -> (-108.9982, 100.0125)
  line L6325 (-108.9982, 80.9625) -> (-103.4989, 90.4875)
  line L6326 (-89.7507, 111.125) -> (-100.7493, 111.125)
  line L6327 (-100.7493, 111.125) -> (-106.2485, 101.6)
  line L6328 (-106.2485, 101.6) -> (-100.7493, 92.075)
  line L6329 (-100.7493, 92.075) -> (-89.7507, 92.075)
  line L6330 (-84.2515, 101.6) -> (-89.7507, 111.125)
  line L6331 (-89.7507, 92.075) -> (-84.2515, 101.6)
  line L6332 (-70.5033, 122.2375) -> (-81.5018, 122.2375)
  line L6333 (-81.5018, 122.2375) -> (-87.0011, 112.7125)
  line L6334 (-87.0011, 112.7125) -> (-81.5018, 103.1875)
  line L6335 (-81.5018, 103.1875) -> (-70.5033, 103.1875)
  line L6336 (-65.0041, 112.7125) -> (-70.5033, 122.2375)
  line L6337 (-70.5033, 103.1875) -> (-65.0041, 112.7125)
  line L6338 (-51.2559, 133.35) -> (-62.2544, 133.35)
  line L6339 (-62.2544, 133.35) -> (-67.7537, 123.825)
  line L6340 (-67.7537, 123.825) -> (-62.2544, 114.3)
  line L6341 (-62.2544, 114.3) -> (-51.2559, 114.3)
  line L6342 (-45.7566, 123.825) -> (-51.2559, 133.35)
  line L6343 (-51.2559, 114.3) -> (-45.7566, 123.825)
  line L6344 (-32.0085, 144.4625) -> (-43.007, 144.4625)
  line L6345 (-43.007, 144.4625) -> (-48.5063, 134.9375)
  line L6346 (-48.5063, 134.9375) -> (-43.007, 125.4125)
  line L6347 (-43.007, 125.4125) -> (-32.0085, 125.4125)
  line L6348 (-26.5092, 134.9375) -> (-32.0085, 144.4625)
  line L6349 (-32.0085, 125.4125) -> (-26.5092, 134.9375)
  line L6350 (-12.7611, 155.575) -> (-23.7596, 155.575)
  line L6351 (-23.7596, 155.575) -> (-29.2589, 146.05)
  line L6352 (-29.2589, 146.05) -> (-23.7596, 136.525)
  line L6353 (-23.7596, 136.525) -> (-12.7611, 136.525)
  line L6354 (-7.2618, 146.05) -> (-12.7611, 155.575)
  line L6355 (-12.7611, 136.525) -> (-7.2618, 146.05)
  line L6356 (6.4863, 166.6875) -> (-4.5122, 166.6875)
  line L6357 (-4.5122, 166.6875) -> (-10.0114, 157.1625)
  line L6358 (-10.0114, 157.1625) -> (-4.5122, 147.6375)
  line L6359 (-4.5122, 147.6375) -> (6.4863, 147.6375)
  line L6360 (11.9856, 157.1625) -> (6.4863, 166.6875)
  line L6361 (6.4863, 147.6375) -> (11.9856, 157.1625)
  line L6362 (25.7337, 177.8) -> (14.7352, 177.8)
  line L6363 (14.7352, 177.8) -> (9.236, 168.275)
  line L6364 (9.236, 168.275) -> (14.7352, 158.75)
  line L6365 (14.7352, 158.75) -> (25.7337, 158.75)
  line L6366 (31.233, 168.275) -> (25.7337, 177.8)
  line L6367 (25.7337, 158.75) -> (31.233, 168.275)
  line L6368 (44.9812, 188.9125) -> (33.9826, 188.9125)
  line L6369 (33.9826, 188.9125) -> (28.4834, 179.3875)
  line L6370 (28.4834, 179.3875) -> (33.9826, 169.8625)
  line L6371 (33.9826, 169.8625) -> (44.9812, 169.8625)
  line L6372 (50.4804, 179.3875) -> (44.9812, 188.9125)
  line L6373 (44.9812, 169.8625) -> (50.4804, 179.3875)
  line L6374 (64.2286, 200.025) -> (53.2301, 200.025)
  line L6375 (53.2301, 200.025) -> (47.7308, 190.5)
  line L6376 (47.7308, 190.5) -> (53.2301, 180.975)
  line L6377 (53.2301, 180.975) -> (64.2286, 180.975)
  line L6378 (69.7278, 190.5) -> (64.2286, 200.025)
  line L6379 (64.2286, 180.975) -> (69.7278, 190.5)
  line L6380 (83.476, 211.1375) -> (72.4775, 211.1375)
  line L6381 (72.4775, 211.1375) -> (66.9782, 201.6125)
  line L6382 (66.9782, 201.6125) -> (72.4775, 192.0875)
  line L6383 (72.4775, 192.0875) -> (83.476, 192.0875)
  line L6384 (88.9753, 201.6125) -> (83.476, 211.1375)
  line L6385 (83.476, 192.0875) -> (88.9753, 201.6125)
  line L6386 (102.7234, 222.25) -> (91.7249, 222.25)
  line L6387 (91.7249, 222.25) -> (86.2256, 212.725)
  line L6388 (86.2256, 212.725) -> (91.7249, 203.2)
  line L6389 (91.7249, 203.2) -> (102.7234, 203.2)
  line L6390 (108.2227, 212.725) -> (102.7234, 222.25)
  line L6391 (102.7234, 203.2) -> (108.2227, 212.725)
  line L6392 (121.9708, 233.3625) -> (110.9723, 233.3625)
  line L6393 (110.9723, 233.3625) -> (105.473, 223.8375)
  line L6394 (105.473, 223.8375) -> (110.9723, 214.3125)
  line L6395 (110.9723, 214.3125) -> (121.9708, 214.3125)
  line L6396 (127.4701, 223.8375) -> (121.9708, 233.3625)
  line L6397 (121.9708, 214.3125) -> (127.4701, 223.8375)
  line L6398 (141.2182, 244.475) -> (130.2197, 244.475)
  line L6399 (130.2197, 244.475) -> (124.7205, 234.95)
  line L6400 (124.7205, 234.95) -> (130.2197, 225.425)
  line L6401 (130.2197, 225.425) -> (141.2182, 225.425)
  line L6402 (146.7175, 234.95) -> (141.2182, 244.475)
  line L6403 (141.2182, 225.425) -> (146.7175, 234.95)
  line L6404 (160.4657, 255.5875) -> (149.4671, 255.5875)
  line L6405 (149.4671, 255.5875) -> (143.9679, 246.0625)
  line L6406 (143.9679, 246.0625) -> (149.4671, 236.5375)
  line L6407 (149.4671, 236.5375) -> (160.4657, 236.5375)
  line L6408 (165.9649, 246.0625) -> (160.4657, 255.5875)
  line L6409 (160.4657, 236.5375) -> (165.9649, 246.0625)
  line L6410 (179.7131, 266.7) -> (168.7145, 266.7)
  line L6411 (168.7145, 266.7) -> (163.2153, 257.175)
  line L6412 (163.2153, 257.175) -> (168.7145, 247.65)
  line L6413 (168.7145, 247.65) -> (179.7131, 247.65)
  line L6414 (185.2123, 257.175) -> (179.7131, 266.7)
  line L6415 (179.7131, 247.65) -> (185.2123, 257.175)
  line L6416 (198.9605, 277.8125) -> (187.962, 277.8125)
  line L6417 (187.962, 277.8125) -> (182.4627, 268.2875)
  line L6418 (182.4627, 268.2875) -> (187.962, 258.7625)
  line L6419 (187.962, 258.7625) -> (198.9605, 258.7625)
  line L6420 (204.4597, 268.2875) -> (198.9605, 277.8125)
  line L6421 (198.9605, 258.7625) -> (204.4597, 268.2875)
  line L6422 (218.2079, 288.925) -> (207.2094, 288.925)
  line L6423 (207.2094, 288.925) -> (201.7101, 279.4)
  line L6424 (201.7101, 279.4) -> (207.2094, 269.875)
  line L6425 (207.2094, 269.875) -> (218.2079, 269.875)
  line L6426 (223.7072, 279.4) -> (218.2079, 288.925)
  line L6427 (218.2079, 269.875) -> (223.7072, 279.4)
  line L6428 (237.4553, 300.0375) -> (226.4568, 300.0375)
  line L6429 (226.4568, 300.0375) -> (220.9575, 290.5125)
  line L6430 (220.9575, 290.5125) -> (226.4568, 280.9875)
  line L6431 (226.4568, 280.9875) -> (237.4553, 280.9875)
  line L6432 (242.9546, 290.5125) -> (237.4553, 300.0375)
  line L6433 (237.4553, 280.9875) -> (242.9546, 290.5125)
  line L6434 (256.7027, 311.15) -> (245.7042, 311.15)
  line L6435 (245.7042, 311.15) -> (240.2049, 301.625)
  line L6436 (240.2049, 301.625) -> (245.7042, 292.1)
  line L6437 (245.7042, 292.1) -> (256.7027, 292.1)
  line L6438 (262.202, 301.625) -> (256.7027, 311.15)
  line L6439 (256.7027, 292.1) -> (262.202, 301.625)
  line L6440 (275.9501, 322.2625) -> (264.9516, 322.2625)
  line L6441 (264.9516, 322.2625) -> (259.4524, 312.7375)
  line L6442 (259.4524, 312.7375) -> (264.9516, 303.2125)
  line L6443 (264.9516, 303.2125) -> (275.9501, 303.2125)
  line L6444 (281.4494, 312.7375) -> (275.9501, 322.2625)
  line L6445 (275.9501, 303.2125) -> (281.4494, 312.7375)
  line L6446 (295.1976, 333.375) -> (284.199, 333.375)
  line L6447 (284.199, 333.375) -> (278.6998, 323.85)
  line L6448 (278.6998, 323.85) -> (284.199, 314.325)
  line L6449 (284.199, 314.325) -> (295.1976, 314.325)
  line L6450 (300.6968, 323.85) -> (295.1976, 333.375)
  line L6451 (295.1976, 314.325) -> (300.6968, 323.85)
  line L6452 (314.445, 344.4875) -> (303.4464, 344.4875)
  line L6453 (303.4464, 344.4875) -> (297.9472, 334.9625)
  line L6454 (297.9472, 334.9625) -> (303.4464, 325.4375)
  line L6455 (303.4464, 325.4375) -> (314.445, 325.4375)
  line L6456 (319.9442, 334.9625) -> (314.445, 344.4875)
  line L6457 (314.445, 325.4375) -> (319.9442, 334.9625)
  line L6458 (333.6924, 355.6) -> (322.6939, 355.6)
  line L6459 (322.6939, 355.6) -> (317.1946, 346.075)
  line L6460 (317.1946, 346.075) -> (322.6939, 336.55)
  line L6461 (322.6939, 336.55) -> (333.6924, 336.55)
  line L6462 (339.1916, 346.075) -> (333.6924, 355.6)
  line L6463 (333.6924, 336.55) -> (339.1916, 346.075)
  line L6464 (352.9398, 366.7125) -> (341.9413, 366.7125)
  line L6465 (341.9413, 366.7125) -> (336.442, 357.1875)
  line L6466 (336.442, 357.1875) -> (341.9413, 347.6625)
  line L6467 (341.9413, 347.6625) -> (352.9398, 347.6625)
  line L6468 (358.4391, 357.1875) -> (352.9398, 366.7125)
  line L6469 (352.9398, 347.6625) -> (358.4391, 357.1875)
  line L6470 (372.1872, 377.825) -> (361.1887, 377.825)
  line L6471 (361.1887, 377.825) -> (355.6894, 368.3)
  line L6472 (355.6894, 368.3) -> (361.1887, 358.775)
  line L6473 (361.1887, 358.775) -> (372.1872, 358.775)
  line L6474 (377.6865, 368.3) -> (372.1872, 377.825)
  line L6475 (372.1872, 358.775) -> (377.6865, 368.3)
  line L6476 (391.4346, 388.9375) -> (380.4361, 388.9375)
  line L6477 (380.4361, 388.9375) -> (374.9368, 379.4125)
  line L6478 (374.9368, 379.4125) -> (380.4361, 369.8875)
  line L6479 (380.4361, 369.8875) -> (391.4346, 369.8875)
  line L6480 (396.9339, 379.4125) -> (391.4346, 388.9375)
  line L6481 (391.4346, 369.8875) -> (396.9339, 379.4125)
  line L6482 (410.682, 400.05) -> (399.6835, 400.05)
  line L6483 (399.6835, 400.05) -> (394.1843, 390.525)
  line L6484 (394.1843, 390.525) -> (399.6835, 381)
  line L6485 (399.6835, 381) -> (410.682, 381)
  line L6486 (416.1813, 390.525) -> (410.682, 400.05)
  line L6487 (410.682, 381) -> (416.1813, 390.525)
  line L6488 (429.9295, 411.1625) -> (418.9309, 411.1625)
  line L6489 (418.9309, 411.1625) -> (413.4317, 401.6375)
  line L6490 (413.4317, 401.6375) -> (418.9309, 392.1125)
  line L6491 (418.9309, 392.1125) -> (429.9295, 392.1125)
  line L6492 (435.4287, 401.6375) -> (429.9295, 411.1625)
  line L6493 (429.9295, 392.1125) -> (435.4287, 401.6375)
  line L6494 (-724.9154, -233.3625) -> (-735.9139, -233.3625)
  line L6495 (-735.9139, -233.3625) -> (-741.4132, -242.8875)
  line L6496 (-741.4132, -242.8875) -> (-735.9139, -252.4125)
  line L6497 (-735.9139, -252.4125) -> (-724.9154, -252.4125)